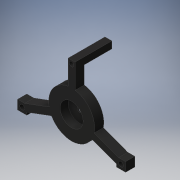
# Autodesk Inventor part: s_mount
Saved by Autodesk Inventor 2016 (Build 200138000, 138)
## iProperties
Created: 2016-09-30
Part Number: s_mount
Material: 一般
Document SubType Name: Modeling
Designer: KOTA-NPC2
Density: 1 g/cm^3
Appearance: ポリカーボネート - クリア(1)
Author: KOTA-NPC2
Autodesk Inventor part; units mm, degrees
ref_plane "YZ Plane" through (0, 0, 0) normal (1, 0, 0) x (0, 1, 0)
ref_plane "XZ Plane" through (0, 0, 0) normal (0, 1, 0) x (-1, 0, 0)
ref_plane "XY Plane" through (0, 0, 0) normal (0, 0, 1) x (1, 0, 0)
sketch "スケッチ1" plane through (0, 0, 0) normal (0, 0, 1) x (1, 0, 0)
  circle A0 centre (0, 27) radius 16 construction
  circle A1 centre (0, 46) radius 1
  line L0 (0, 60.4716) -> (0, -64.9114) construction
  circle A2 centre (0, 27) radius 15 construction
  line L1 (1.5, 47.5) -> (-1.5, 47.5)
  line L2 (-1.5, 47.5) -> (-1.5, 44.5)
  line L3 (-1.5, 44.5) -> (1.5, 44.5)
  line L4 (1.5, 44.5) -> (1.5, 47.5)
  line L5 (1.5, 44.5) -> (1.5, 42.9295)
  line L6 (-1.5, 44.5) -> (-1.5, 42.9295)
  circle A3 centre (21.5, 19) radius 1.5 construction
  circle A4 centre (-21.5, 19) radius 1.5 construction
  line L7 (0, 27) -> (21.5, 19) construction
  line L8 (0, 27) -> (-21.5, 19) construction
  circle A5 centre (0, 27) radius 10
  circle A6 centre (0, 27) radius 5
  line L9 (-1.5, 44.5) -> (-1.5, 36.8869)
  line L10 (1.5, 44.5) -> (1.5, 36.8869)
  line L11 (-22.0231, 20.4058) -> (-9.7893, 24.958) construction
  line L12 (-20.9769, 17.5942) -> (-8.7431, 22.1463) construction
  line L13 (22.0231, 20.4058) -> (9.7893, 24.958) construction
  line L14 (20.9769, 17.5942) -> (8.7431, 22.1463) construction
  circle A7 centre (0, 27) radius 1
  circle A8 centre (21.5, 19) radius 1.05
  circle A9 centre (-21.5, 19) radius 1.05
  line L15 (19.5, 21) -> (23.5, 21) construction
  line L16 (23.5, 21) -> (23.5, 17) construction
  line L17 (23.5, 17) -> (19.5, 17) construction
  line L18 (19.5, 17) -> (19.5, 21) construction
  line L19 (19.5, 21) -> (23.5, 17) construction
  line L20 (23.5, 21) -> (19.5, 17) construction
  line L21 (9.7893, 24.958) -> (20.4263, 21)
  line L22 (20.4263, 21) -> (23.5, 21)
  line L23 (23.5, 21) -> (23.5, 17)
  line L24 (23.5, 17) -> (19.5, 17)
  line L25 (19.5, 17) -> (19.5, 18.1437)
  line L26 (19.5, 18.1437) -> (8.7431, 22.1463)
  line L27 (-23.5, 17) -> (-19.5, 17) construction
  line L28 (-19.5, 17) -> (-19.5, 21) construction
  line L29 (-19.5, 21) -> (-23.5, 21) construction
  line L30 (-23.5, 21) -> (-23.5, 17) construction
  line L31 (-23.5, 17) -> (-19.5, 21) construction
  line L32 (-19.5, 17) -> (-23.5, 21) construction
  line L33 (-9.7893, 24.958) -> (-20.4263, 21)
  line L34 (-20.4263, 21) -> (-23.5, 21)
  line L35 (-23.5, 21) -> (-23.5, 17)
  line L36 (-23.5, 17) -> (-19.5, 17)
  line L37 (-19.5, 17) -> (-19.5, 18.1437)
  line L38 (-19.5, 18.1437) -> (-8.7431, 22.1463)
  line L39 (-40.2847, 27) -> (38.7153, 27) construction
  point P0 (0, 0)
  dimension "d0" = 32
  dimension "d1" = 2
  dimension "d3" = 27
  dimension "d4" = 30
  dimension "d5" = 3
  dimension "d6" = 3
  dimension "d8" = 1.5
  dimension "d15" = 20
  dimension "d16" = 10
  dimension "d20" = 2
  dimension "d29" = 27
  dimension "d30" = 27
  dimension "d32" = 3
  dimension "d33" = 3
  dimension "d35" = 2.1
  dimension "d36" = 2.1
  dimension "d40" = 4
  dimension "d41" = 4
  dimension "d42" = 4
  dimension "d43" = 4
  dimension "d48" = 19
  dimension "d49" = 1.5
  dimension "d50" = 21.5
  dimension "d51" = 21.5
  constraints: 80 end point, 12 parallel, 12 point on circle, 11 point on line, 10 centre point, 6 coincident, 6 perpendicular, 5 collinear, 4 horizontal, 4 midpoint, 4 tangent, 3 vertical, 2 other
  measures "d0" diameter of A0
  measures "d1" diameter of A1
  measures "d3" distance of point (0, 0) A0.centre
  measures "d4" diameter of A2
  measures "d5" distance of L1.start L1.end
  measures "d6" distance of L3.end L1.start
  measures "d8" distance between parallel lines of L0 L4
  measures "d15" diameter of A5
  measures "d16" diameter of A6
  measures "d20" diameter of A7
  measures "d29" vertical distance of L8.end A1.centre
  measures "d30" vertical distance of A1.centre L7.end
  measures "d32" diameter of A4
  measures "d33" diameter of A3
  measures "d35" diameter of A9
  measures "d36" diameter of A8
  measures "d40" distance of L15.end L16.end
  measures "d41" distance of L16.end L17.end
  measures "d42" distance of L29.end L28.end
  measures "d43" distance of L28.end L27.end
  measures "d48" distance from line of L39 A1.centre
  measures "d49" distance from line of A1.centre L3
  measures "d50" distance from line of L0 L7.end
  measures "d51" distance from line of L0 L8.end
extrude "押し出し1" add sketch "スケッチ1" against normal blind 16 contours A1 | L4 L3 L2 L1
extrude "押し出し3" cut sketch "スケッチ1" against normal blind 4 contours A1
sketch "スケッチ6" plane through (0, 0, 0) normal (0, 0, 1) x (1, 0, 0)
  circle A0 centre (0, 27) radius 5 projected
  circle A1 centre (0, 27) radius 5
  point P0 (0, 0)
  dimension "d23" = 10
  constraints: 1 centre point, 1 coincident
  measures "d23" diameter of A1
sketch "スケッチ7" plane through (0, 0, -16) normal (0, 0, -1) x (-1, 0, 0)
  circle A0 centre (0, 46) radius 1 projected
  point P0 (0, 0)
extrude "押し出し7" cut sketch "スケッチ7" against normal blind 3.5
extrude "押し出し9" add sketch "スケッチ1" against normal blind 4 contours L5 L10 A5 L9 L6 L3 | A5 | A5 L38 L37 L36 L35 L34 L33 | L21 L22 L23 L24 L25 L26 A5 | A6
extrude "押し出し10" cut sketch "スケッチ6" against normal blind 3.5
sketch "スケッチ8" plane through (0, 0, 0) normal (0, 0, 1) x (1, 0, 0)
  circle A0 centre (0, 27) radius 5 projected
  circle A1 centre (21.5, 19) radius 1.05 projected
  circle A2 centre (-21.5, 19) radius 1.05 projected
  circle A3 centre (0, 46) radius 1 projected
  line L0 (1.5, 47.5) -> (-1.5, 47.5) projected
  line L1 (-1.5, 47.5) -> (-1.5, 36.8869) projected
  arc A4 (-1.5, 36.8869) -> (-9.7893, 24.958) centre (0, 27) ccw projected
  line L2 (-9.7893, 24.958) -> (-20.4263, 21) projected
  line L3 (-20.4263, 21) -> (-23.5, 21) projected
  line L4 (-23.5, 21) -> (-23.5, 17) projected
  line L5 (-23.5, 17) -> (-19.5, 17) projected
  line L6 (-19.5, 17) -> (-19.5, 18.1437) projected
  line L7 (-19.5, 18.1437) -> (-8.7431, 22.1463) projected
  arc A5 (-8.7431, 22.1463) -> (8.7431, 22.1463) centre (0, 27) ccw projected
  line L8 (8.7431, 22.1463) -> (19.5, 18.1437) projected
  line L9 (19.5, 18.1437) -> (19.5, 17) projected
  line L10 (19.5, 17) -> (23.5, 17) projected
  line L11 (23.5, 17) -> (23.5, 21) projected
  line L12 (23.5, 21) -> (20.4263, 21) projected
  line L13 (20.4263, 21) -> (9.7893, 24.958) projected
  arc A6 (9.7893, 24.958) -> (1.5, 36.8869) centre (0, 27) ccw projected
  line L14 (1.5, 36.8869) -> (1.5, 47.5) projected
  circle A7 centre (0, 27) radius 1 projected
  point P0 (0, 0)
equation "\"d30\" = d29"
equation "\"d33\" = d32"
equation "\"d36\" = d35"
equation "\"d41\" = d40"
equation "\"d42\" = d40"
equation "\"d43\" = d40"
equation "\"d51\" = d50"
